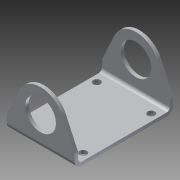
# Autodesk Inventor part: Bearing Mount 5
Saved by Autodesk Inventor 2013 (Build 170138000, 138)
## iProperties
Created: 2013-01-18
Part Number: Bearing Mount 5
Material: Aluminum 6061
Document SubType Name: Sheet Metal
Designer: actoennies
Density: 2.71 g/cm^3
Sheet Metal Rule: Default
Mass: 75.1773 g
Surface Area: 196.673 cm^2
Volume: 27.7407 cm^3
Author: actoennies
Autodesk Inventor part; units mm, degrees
ref_plane "YZ Plane" through (0, 0, 0) normal (1, 0, 0) x (0, 1, 0)
ref_plane "XZ Plane" through (0, 0, 0) normal (0, 1, 0) x (-1, 0, 0)
ref_plane "XY Plane" through (0, 0, 0) normal (0, 0, 1) x (1, 0, 0)
sketch "Sketch1" plane through (0, 0, 0) normal (0, 1, 0) x (-1, 0, 0)
  line L0 (0, 0) -> (63.5, 0)
  line L1 (63.5, 0) -> (63.5, 92.1004)
  line L2 (63.5, 92.1004) -> (0, 92.1004)
  line L3 (0, 92.1004) -> (0, 0)
  dimension "d0" = 92.1004
  dimension "d2" = 63.5
  measures "d0" distance between parallel lines of L0 L2
  measures "d2" distance of L1.end L2.end
extrude "Plate1" add sketch "Sketch1" along normal blind 3.175
sketch "Sketch2" plane through (0, 0, 88.9254) normal (0, 0, 1) x (1, 0, 0)
  line L0 (-63.5, 0) -> (0, 0)
  line L1 (0, 0) -> (0, 50.8)
  line L2 (0, 50.8) -> (-63.5, 50.8)
  line L3 (-63.5, 50.8) -> (-63.5, 0)
  constraints: 6 end point, 1 horizontal, 1 perpendicular, 1 vertical
edge flange "Flange1" height 50.8 angle 90 thickness 3.175 bend radius 3.175 thickness toward (0, 0, 1) relief tear relief width 3.175 relief depth 1.5875 corner gap 3.175 corner form 0 edges at (-31.75, 3.175, 92.1004) (-31.75, 3.175, 0) wall of the first edge with corners at (-63.5, 0, 88.9254) (0, 0, 88.9254) (0, 50.8, 88.9254) (-63.5, 50.8, 88.9254)
bend "Bend1"
corner "Corner1"
sketch "Sketch3" plane through (-63.5, 50.8, 92.1004) normal (0, 0, 1) x (1, 0, 0)
  line L0 (0, -44.45) -> (63.5, -44.45) projected
  line L1 (63.5, 0) -> (63.5, -44.45) projected
  line L2 (0, 0) -> (63.5, 0) projected
  line L3 (0, -44.45) -> (0, 0) projected
  circle A0 centre (31.75, -22.225) radius 14.2875
  arc A1 (51.9461, -12.9478) -> (11.5539, -12.9478) centre (31.75, -22.225) ccw
  line L4 (0, -38.1) -> (11.5539, -12.9478)
  line L5 (51.9461, -12.9478) -> (63.5, -38.1)
  point P0 (63.5, -50.8)
  dimension "d14" = 28.575
  dimension "d15" = 6.35
  dimension "d16" = 28.575
  dimension "d17" = 44.45
  dimension "d18" = 31.75
  dimension "d19" = 6.35
  constraints: 4 end point, 2 centre point, 2 point on circle, 2 point on line, 2 tangent, 1 coincident
  measures "d14" diameter of A0
  measures "d15" distance of L0.end L5.end
  measures "d16" vertical distance of A0.centre point (63.5, -50.8)
  measures "d17" diameter of A1
  measures "d18" distance from line of L1 A0.centre
  measures "d19" distance from line of L4.start L0
extrude "Cut1" cut sketch "Sketch3" against normal blind 2540 contours L3 L2 A1 L4 | L5 A1 L2 L1 | A0
sketch "Sketch4" plane through (0, 0, 0) normal (0, -1, 0) x (1, 0, 0)
  line L0 (0, 85.7504) -> (0, 6.35) projected
  line L1 (-63.5, 6.35) -> (-63.5, 85.7504) projected
  circle A0 centre (-57.15, 77.8002) radius 3.3782
  circle A1 centre (-6.35, 77.8002) radius 3.3782
  circle A2 centre (-57.15, 14.3002) radius 3.3782
  circle A3 centre (-6.35, 14.3002) radius 3.3782
  line L2 (-63.5, 46.0502) -> (0, 46.0502)
  point P0 (0, 0)
  dimension "d22" = 6.7564
  dimension "d23" = 6.7564
  dimension "d24" = 6.7564
  dimension "d25" = 6.7564
  dimension "d26" = 31.75
  dimension "d27" = 31.75
  dimension "d28" = 31.75
  dimension "d29" = 31.75
  dimension "d30" = 6.35
  dimension "d31" = 6.35
  dimension "d32" = 6.35
  dimension "d33" = 6.35
  constraints: 4 centre point, 2 end point, 2 midpoint
  measures "d22" diameter of A0
  measures "d23" diameter of A1
  measures "d24" diameter of A2
  measures "d25" diameter of A3
  measures "d26" distance from line of L2 A3.centre
  measures "d27" distance from line of L2 A2.centre
  measures "d28" distance from line of L2 A0.centre
  measures "d29" distance from line of L2 A1.centre
  measures "d30" distance from line of L0 A1.centre
  measures "d31" distance from line of L0 A3.centre
  measures "d32" distance from line of L1 A2.centre
  measures "d33" distance from line of L1 A0.centre
extrude "Cut2" cut sketch "Sketch4" against normal blind 3.175
equation "\"d34\" = Thickness"
equation "\"d4\" = BendReliefWidth"
equation "\"d5\" = BendReliefDepth"
equation "\"d6\" = MinimumRemnant"
equation "\"d7\" = BendRadius"
equation "\"d10\" = BendRadius"
equation "\"d11\" = CornerReliefSize"
equation "\"d12\" = GapSize"
equation "\"d13\" = JacobiRadiusSize"
equation "\"BendRadius\" = Thickness"
equation "\"BendReliefWidth\" = Thickness"
equation "\"BendReliefDepth\" = 0.5 * Thickness"
equation "\"CornerReliefSize\" = 4 * Thickness"
equation "\"MinimumRemnant\" = 2 * Thickness"
equation "\"TransitionRadius\" = BendRadius"
equation "\"JacobiRadiusSize\" = BendRadius"
equation "\"GapSize\" = Thickness"
equation "\"d3\" = BendRadius"
equation "\"Thickness\" = 3.175"
body "Solid1"
